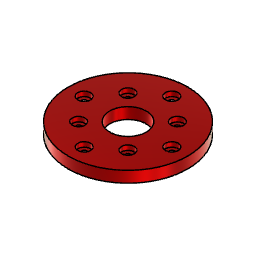
Braço robótico 3.0(Tampa da base) v10 (Autodesk Fusion 360 design; units mm, degrees)
Autodesk Fusion 360 part; units mm, degrees
sketch "Sketch1" plane through (0, 0, 0) normal (0, 0, 1) x (1, 0, 0)
  circle A0 centre (0, 0) radius 37.5
  dimension "d1" = 75
  constraint coincident A0.centre origin
  measures "d1" diameter of A0
extrude "Extrude1" add sketch "Sketch1" along normal blind 7
sketch "Sketch2" plane through (0, 0, 7) normal (0, 0, 1) x (-1, 0, 0)
  circle A0 centre (0, 0) radius 37.5
  circle A1 centre (0, 0) radius 11.493
  dimension "d4" = 22.986
  constraint concentric A0 A1
  measures "d4" diameter of A1
extrude "Extrude2" cut sketch "Sketch2" against normal blind 13 contours A1
sketch "Sketch3" plane through (0, 0, 7) normal (0, 0, 1) x (-1, 0, 0)
  circle A0 centre (0, 0) radius 11.493
  circle A1 centre (0, 0) radius 37.5
  line L0 (0, 0) -> (-15.4998, -15.4998)
  line L1 (0, 0) -> (15.4998, -15.4998)
  line L2 (0, 0) -> (15.4998, 15.4998)
  line L3 (0, 0) -> (-15.4998, 15.4998)
  line L4 (-0.0074, 37.5) -> (-0.0074, 26.5)
  line L5 (-37.5, -0.0074) -> (-26.5, -0.0074)
  line L6 (0.0074, -37.5) -> (0.0074, -26.5)
  line L7 (37.5, 0.0074) -> (26.5, 0.0074)
  dimension "d10" = 11
  dimension "d12" = 360
  constraint coincident A1 L4.start
  constraint vertical L4
  measures "d10" distance of L4.start L4.end
hole "Hole1" at (15.4998, 15.4998, 7) at (15.4998, -15.4998, 7) at (-15.4998, -15.4998, 7) at (-15.4998, 15.4998, 7) direction (0, 0, -1) diameter 3.332 end through all counterbore diameter 8 counterbore depth 3
sketch "Sketch4" plane through (0, 0, 7) normal (0, 0, 1) x (-1, 0, 0)
  circle A0 centre (15.4998, 15.4998) radius 4
  circle A1 centre (-15.4998, -15.4998) radius 4
  circle A2 centre (-15.4998, 15.4998) radius 4
  circle A3 centre (15.4998, -15.4998) radius 4
  circle A4 centre (0, 0) radius 11.493
  circle A5 centre (0, 0) radius 37.5
  line L0 (0, 37.5) -> (0, 27.5)
  line L1 (-37.5, 0) -> (-27.5, 0)
  line L2 (0, -37.5) -> (0, -27.5)
  line L3 (37.5, 0) -> (27.5, 0)
  dimension "d22" = 10
  dimension "d24" = 360
  constraint coincident A5 L0.start
  measures "d22" distance of L0.start L0.end
hole "Hole2" at (-27.5, 0, 7) at (0, 27.5, 7) at (27.5, 0, 7) at (0, -27.5, 7) direction (0, 0, -1) diameter 3.332 depth 50 tip angle 180 counterbore diameter 8 counterbore depth 3
thread "Thread2" "ISO Metric profile 4.0 M4x0.7 6H"
component "6627T91_Stepper Motor" placed x (1, 0, 0) y (0, 1, 0) z (0, 0, 1) at (0, 0, 0)
component "7965K17_Multipurpose Sleeve Bearing with Groove" placed x (1, 0, 0) y (0, 1, 0) z (0, 0, 1) at (0, 0, 0)
